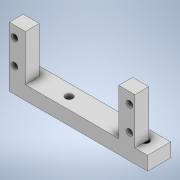
# Autodesk Inventor part: vydacha_3
Saved by Autodesk Inventor 2020 (Build 240168000, 168)
## iProperties
Created: 2022-07-27
Part Number: vydacha_3
Material: Типовые
Document SubType Name: Modeling
Designer: akapu
Density: 1 g/cm^3
Appearance: По умолчанию
Author: akapu
Autodesk Inventor part; units mm, degrees
ref_plane "YZ Plane" through (0, 0, 0) normal (1, 0, 0) x (0, 1, 0)
ref_plane "XZ Plane" through (0, 0, 0) normal (0, 1, 0) x (-1, 0, 0)
ref_plane "XY Plane" through (0, 0, 0) normal (0, 0, 1) x (1, 0, 0)
sketch "Эскиз2" plane through (0, 0, 0) normal (0, 0, 1) x (1, 0, 0)
  line L0 (0, 0) -> (40.5, 0)
  line L1 (40.5, 0) -> (40.5, -20)
  line L2 (40.5, -20) -> (0, -20)
  line L3 (0, -20) -> (0, 0)
  line L4 (40.5, 0) -> (40.5, -4.7)
  line L5 (40.5, -4.7) -> (45.2, -4.7)
  line L6 (45.2, -15.3) -> (40.5, -15.3)
  line L7 (40.5, -15.3) -> (40.5, -20)
  line L8 (0, -4.7) -> (-4.7, -4.7)
  line L9 (-4.7, -15.3) -> (0, -15.3)
  line L10 (0, 0) -> (-7, 0)
  line L11 (-7, 0) -> (-7, -20)
  line L12 (-7, -20) -> (40.5, -20)
  line L13 (40.5, -20) -> (47.5, -20)
  line L14 (47.5, -20) -> (47.5, 0)
  line L15 (47.5, 0) -> (40.5, 0)
  circle A0 centre (-4.7, -4.7) radius 1.4
  circle A1 centre (-4.7, -15.3) radius 1.4
  circle A2 centre (45.2, -4.7) radius 1.4
  circle A3 centre (45.2, -15.3) radius 1.4
  dimension "d9" = 40.5
  dimension "d11" = 4.7
  dimension "d12" = 4.7
  dimension "d14" = 4.7
  dimension "d15" = 7
  dimension "d16" = 7
  dimension "d17" = 2.8
  dimension "d18" = 2.8
  dimension "d19" = 2.8
  dimension "d20" = 2.8
  constraints: 32 end point, 6 perpendicular, 6 point on line, 4 centre point, 4 coincident, 2 horizontal, 2 parallel, 1 collinear
  measures "d9" distance of L1.end L2.end
  measures "d11" distance of L0.end L4.end
  measures "d12" distance of L4.end L5.end
  measures "d14" distance of L8.start L8.end
  measures "d15" distance of L0.start L10.end
  measures "d16" distance of L1.end L13.end
  measures "d17" diameter of A0
  measures "d18" diameter of A1
  measures "d19" diameter of A2
  measures "d20" diameter of A3
extrude "Выдавливание2" add sketch "Эскиз2" along normal blind 6 contours L3 L12 L11 L10 | L15 L14 L13 L1
sketch "Эскиз3" plane through (-7, -20, 0) normal (0, -1, 0) x (1, 0, 0)
  line L0 (7, 6) -> (0, 6) projected
  line L1 (47.5, 0) -> (54.5, 0) projected
  line L2 (0, 6) -> (54.5, 6)
  line L3 (54.5, 6) -> (54.5, 0)
  line L4 (54.5, 0) -> (0, 0)
  line L5 (0, 0) -> (0, 6)
  line L6 (47.5, 0) -> (47.5, 6) projected
  line L7 (47.5, 6) -> (37.5, 6)
  line L8 (37.5, 6) -> (54.0635, 6)
  line L9 (54.0635, 6) -> (20.9365, 6)
  line L10 (20.9365, 6) -> (20.9365, 1)
  line L11 (20.9365, 1) -> (54.0635, 1)
  line L12 (54.0635, 1) -> (54.0635, 6)
  circle A0 centre (20.9365, 1) radius 1.6
  circle A1 centre (54.0635, 1) radius 1.6
  line L13 (0, 6) -> (60, 6)
  line L14 (60, 6) -> (60, -4)
  line L15 (60, -4) -> (0, -4)
  line L16 (0, -4) -> (0, 6)
  point P0 (7, 0)
  point P1 (0, 0)
  dimension "d23" = 10
  dimension "d24" = 16.5635
  dimension "d25" = 33.127
  dimension "d26" = 5
  dimension "d27" = 3.2
  dimension "d28" = 3.2
  dimension "d29" = 60
  dimension "d30" = 10
  constraints: 28 end point, 4 parallel, 4 perpendicular, 3 point on line, 2 centre point, 2 coincident, 2 horizontal, 1 vertical
  measures "d23" distance of L6.end L7.end
  measures "d24" distance of L7.end L8.end
  measures "d25" distance of L8.end L9.end
  measures "d26" distance of L9.end L10.end
  measures "d27" diameter of A0
  measures "d28" diameter of A1
  measures "d29" distance of L14.end L15.end
  measures "d30" distance of L13.end L14.end
extrude "Выдавливание3" add sketch "Эскиз3" along normal blind 6 contours L2 L10 A0 L4 L5 L0 | L2 L6 L11 A0 L10 | L4 A0 L1 A1 L3 L13 L14 L15 L16 | L2 L12 A1 L11 L6 | L11 L6 L4 A0 | L2 L3 A1 L12 | L11 A1 L1 L6
